frame8000f120 (Autodesk Fusion 360 design; units mm, degrees)
Autodesk Fusion 360 part; units mm, degrees
sketch "Sketch1" plane through (0, 0, 0) normal (0, 0, 1) x (1, 0, 0)
  line L0 (50, -75) -> (-50, -75)
  line L1 (-50, -75) -> (-50, 75)
  line L2 (-50, 75) -> (50, 75)
  line L3 (50, 75) -> (50, -75)
  line L4 (50, -75) -> (-50, 75) construction
  line L5 (-50, -75) -> (50, 75) construction
  line L6 (9.5, 77.5) -> (-9.5, 77.5)
  line L7 (-9.5, 77.5) -> (-9.5, 75)
  line L8 (9.5, 75) -> (9.5, 77.5)
  line L9 (9.5, 77.5) -> (-9.5, 72.5) construction
  line L10 (-9.5, 77.5) -> (9.5, 72.5) construction
  line L11 (-33.5, 50) -> (33.5, 50)
  line L12 (-33.5, 40.1) -> (33.5, 40.1)
  line L13 (-33.5, 50) -> (-33.5, 40.1)
  line L14 (33.5, 50) -> (33.5, 40.1)
  line L15 (-50, 30.8) -> (50, 30.8)
  line L16 (-33.5, 50) -> (-33.5, 40.1)
  line L17 (33.5, 50) -> (33.5, 40.1)
  line L18 (-50, -70) -> (50, -70)
  line L19 (-30.95, 30.8) -> (-30.95, -70)
  line L20 (0, 30) -> (0, -70)
  line L21 (30.95, 30.8) -> (30.95, -70)
  line L22 (-30, 30.8) -> (-30, -70)
  line L23 (30, 30.8) -> (30, -70)
  line L24 (-30, 26.8) -> (30, 26.8)
  line L25 (-30, -66) -> (30, -66)
  point P0 (0, 75)
  dimension "d1" = 100
  dimension "d2" = 150
  dimension "d3" = 19
  dimension "d4" = 5
  dimension "d5" = 25
  dimension "d6" = 9.9
  dimension "d8" = 9.3
  dimension "d9" = 5
  dimension "d10" = 30.95
  dimension "d11" = 30
  dimension "d12" = 4
  dimension "d13" = 4
  constraint horizontal L0
  constraint perpendicular L0 L1
  constraint parallel L0 L2
  constraint parallel L1 L3
  constraint coincident L4 origin
  constraint coincident L5 origin
  constraint horizontal L6
  constraint perpendicular L6 L7
  constraint parallel L7 L8
  constraint coincident L9 P0
  constraint coincident L10 P0
  constraint midpoint L2 P0
  constraint coincident L2 L7.end
  constraint coincident L2 L8.start
  constraint perpendicular L1 L11
  constraint perpendicular L3 L12
  constraint perpendicular L12 L13
  constraint coincident L1 L15.start
  constraint coincident L3 L15.end
  constraint perpendicular L3 L15
  constraint perpendicular L12 L17
  constraint coincident L1 L18.start
  constraint coincident L3 L18.end
  constraint perpendicular L3 L18
  constraint coincident L15 L19.start
  constraint coincident L18 L19.end
  constraint perpendicular L18 L19
  constraint midpoint L18 L20.end
  constraint perpendicular L18 L20
  constraint symmetric L19.start L20 L21.start
  constraint symmetric L19.end L20 L21.end
  constraint coincident L15 L22.start
  constraint coincident L18 L22.end
  constraint perpendicular L18 L22
  constraint symmetric L20 L22.start L23.start
  constraint symmetric L20 L22.end L23.end
  constraint coincident L22 L24.start
  constraint perpendicular L20 L24
  constraint coincident L22 L25.start
  constraint perpendicular L22 L25
  measures "d1" distance of L1.end L2.end
  measures "d2" distance of L0.end L1.end
  measures "d3" distance of L9.end L10.end
  measures "d4" distance of L6.end L9.end
  measures "d5" distance of L2 L11
  measures "d6" distance of L11 L12
  measures "d8" distance of L12 L15
  measures "d9" distance of L0 L18
  measures "d10" distance of origin L19
  measures "d11" distance of L20 L22
  measures "d12" distance of L15 L24
  measures "d13" distance of L18 L25
extrude "Extrude1" add sketch "Sketch1" along normal blind 3.4 contours L0 L1 L3 L18 | L3 L15 L18 L21 | L1 L15 L18 L19 | L1 L2 L3 L15 | L2 L6 L7 L8 makes body 1
extrude "Extrude2" add sketch "Sketch1" along normal blind 0.8 separate body contours L15 L18 L21 L23 | L15 L18 L19 L22 | L18 L20 L23 L25 | L18 L20 L22 L25 | L15 L22 L23 L24 makes body 2
fillet "Fillet1" radius 2 6 edges at (50, 75, 1.7) (-50, 75, 1.7) (-9.5, 77.5, 1.7) (9.5, 77.5, 1.7) (-50, -75, 1.7) (50, -75, 1.7) on bodies 1
fillet "Fillet2" radius 1 4 edges at (33.5, 40.1, 1.7) (33.5, 50, 1.7) (-33.5, 50, 1.7) (-33.5, 40.1, 1.7) on bodies 1
extrude "Extrude3" cut sketch "Sketch1" along normal blind 1.5 contours L2 L6 L7 L8 bodies 1
